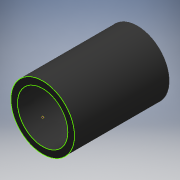
# Autodesk Inventor part: DPLX_P012_Rubber_Insert_Transformer
Saved by Autodesk Inventor 2018 (Build 220112000, 112)
## iProperties
Created: 2018-06-08
Part Number: DPLX_P012_Rubber_Insert_Transformer
Material: Generic
Document SubType Name: Modeling
Designer: DPLXuser
Density: 1 g/cm^3
Appearance: Rubber - Black
Author: DPLXuser
Autodesk Inventor part; units mm, degrees
ref_plane "YZ Plane" through (0, 0, 0) normal (1, 0, 0) x (0, 1, 0)
ref_plane "XZ Plane" through (0, 0, 0) normal (0, 1, 0) x (-1, 0, 0)
ref_plane "XY Plane" through (0, 0, 0) normal (0, 0, 1) x (1, 0, 0)
sketch "Sketch1" plane through (0, 0, 0) normal (0, 1, 0) x (-1, 0, 0)
  circle A0 centre (0, 0) radius 5.6115
  circle A1 centre (0, 0) radius 4.445
  dimension "d0" = 11.223
  dimension "d1" = 8.89
  constraints: 2 centre point, 2 coincident
  measures "d0" diameter of A0
  measures "d1" diameter of A1
extrude "Extrusion1" add sketch "Sketch1" along normal blind 16.764
sketch "Sketch2" plane through (0, 0, 0) normal (0, -1, 0) x (1, 0, 0)
  point P0 (0, 0)
sketch "Sketch3" plane through (0, 0, 0) normal (0, -1, 0) x (1, 0, 0)
  circle A0 centre (0, 0) radius 5.6115 projected
  circle A1 centre (0, 0) radius 5.6115
  circle A2 centre (0, 0) radius 4.445
  constraints: 2 centre point, 2 coincident
body "Solid1"
